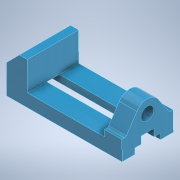
# Autodesk Inventor part: Parte2_Base
Saved by Autodesk Inventor 2021 (Build 250183000, 183)
## iProperties
Created: 2020-10-13
Part Number: Parte2_Base
Material: Steel, Carbon
Document SubType Name: Modeling
Designer: Alejandro Guevara
Density: 7.85 g/cm^3
Appearance: Sky Blue Dark
Author: Alejandro Guevara
Autodesk Inventor part; units mm, degrees
ref_plane "YZ Plane" through (0, 0, 0) normal (1, 0, 0) x (0, 1, 0)
ref_plane "XZ Plane" through (0, 0, 0) normal (0, 1, 0) x (-1, 0, 0)
ref_plane "XY Plane" through (0, 0, 0) normal (0, 0, 1) x (1, 0, 0)
sketch "Sketch1" plane through (0, 0, 0) normal (0, 0, 1) x (1, 0, 0)
  line L0 (-71.9595, -8.3565) -> (72.0387, -7.6433)
  line L1 (72.0387, -7.6433) -> (71.7812, 44.356)
  line L2 (71.7812, 44.356) -> (49.7815, 44.2471)
  line L3 (49.7815, 44.2471) -> (49.9598, 8.2475)
  line L4 (49.9598, 8.2475) -> (-46.0391, 7.7721)
  line L5 (-46.0391, 7.7721) -> (-46.2173, 43.7717)
  line L6 (-46.2173, 43.7717) -> (-56.2172, 43.7221)
  line L7 (-71.9595, -8.3565) -> (-71.9595, 27.7497)
  line L8 (-71.9595, 27.7497) -> (-56.2172, 43.7221)
  point P0 (0, 0)
  dimension "d0" = 144
  dimension "d1" = 52
  dimension "d2" = 22
  dimension "d3" = 36
  dimension "d4" = 96
  dimension "d5" = 36
  dimension "d6" = 10
  dimension "d8" = 72
  dimension "d9" = 16
  dimension "d10" = 8
  constraints: 18 end point, 4 perpendicular, 2 point on line, 1 vertical
  measures "d0" distance of L0.start L0.end
  measures "d1" distance of L0.end L1.end
  measures "d2" distance of L1.end L2.end
  measures "d3" distance of L2.end L3.end
  measures "d4" distance of L3.end L4.end
  measures "d5" distance of L4.end L5.end
  measures "d6" distance of L5.end L6.end
  measures "d8" distance from line of L1 point (0, 0)
  measures "d9" distance between parallel lines of L0 L4
  measures "d10" distance from line of L4 point (0, 0)
extrude "Extrusion1" add sketch "Sketch1" along normal blind 64
sketch "Sketch3" plane through (71.7812, 44.356, 64) normal (0.9999877, 0.0049523, 0) x (0, 0, -1)
  line L0 (64, -52) -> (64, 0) projected
  line L1 (0, -52) -> (0, 0) projected
  line L2 (48, -52) -> (48, -45)
  line L3 (40, -45) -> (40, -36)
  line L4 (48, -45) -> (40, -45)
  line L5 (40, -36) -> (32, -36)
  line L6 (64, -36) -> (0, -36) projected
  line L7 (16, -52) -> (16, -45)
  line L8 (24, -45) -> (24, -36)
  line L9 (16, -45) -> (24, -45)
  line L10 (24, -36) -> (32, -36)
  line L11 (16, -52) -> (48, -52)
  line L12 (64, -52) -> (0, -52) projected
  line L13 (64, -36) -> (64, 0) projected
  arc A0 (58.5136, -26.6786) -> (61, -28) centre (61, -25) ccw
  arc A1 (45.2611, -7.0477) -> (18.7389, -7.0477) centre (32, -16) ccw
  circle A2 centre (32, -16) radius 8
  line L14 (64, 0) -> (0, 0) projected
  line L15 (45.2611, -7.0477) -> (58.5136, -26.6786)
  line L16 (64, -28) -> (61, -28)
  line L17 (64, -15.8943) -> (0, -15.8943) projected
  arc A3 (3, -28) -> (5.4864, -26.6786) centre (3, -25) ccw
  line L18 (18.7389, -7.0477) -> (5.4864, -26.6786)
  line L19 (0, -28) -> (3, -28)
  line L20 (0, -36) -> (0, 0) projected
  line L21 (0, -28) -> (0, 0)
  line L22 (64, 0) -> (0, 0) projected
  line L23 (0, 0) -> (64, 0)
  line L24 (64, 0) -> (64, -28)
  point P0 (64, -44)
  point P1 (32, 0)
  point P2 (0, -28)
  point P3 (64, -28)
  dimension "d13" = 64
  dimension "d16" = 7
  dimension "d18" = 32
  dimension "d19" = 16
  dimension "d20" = 16
  dimension "d21" = 9
  dimension "d24" = 24
  dimension "d26" = 6
  dimension "d27" = 32
  dimension "d28" = 16
  dimension "d29" = 32
  dimension "d30" = 64
  constraints: 32 end point, 6 point on circle, 5 tangent, 4 centre point, 4 perpendicular, 2 collinear, 1 coincident, 1 midpoint, 1 point on line
  measures "d13" distance between parallel lines of L0 L1
  measures "d16" distance of L2.start L2.end
  measures "d18" distance between parallel lines of L2 L7
  measures "d19" distance between parallel lines of L3 L8
  measures "d20" distance from line of L0.start L2
  measures "d21" distance between parallel lines of L6 L9
  measures "d24" distance of L0.start L16.start
  measures "d26" diameter of A0
  measures "d27" diameter of A1
  measures "d28" diameter of A2
  measures "d29" distance from line of L1 A2.centre
  measures "d30" distance between parallel lines of L13 L1
extrude "Extrusion2" cut sketch "Sketch3" against normal through all contours L11 L7 L9 L8 L6 L5 L3 L4 L2
extrude "Extrusion3" cut sketch "Sketch3" against normal blind 22 contours L16 A0 L15 L17 L0 | L17 L15 A1 L14 L0 | A1 L18 L17 L1 L14 | L17 A2 | A2 L17 | L1 L17 L18 A3 L19
sketch "Sketch4" plane through (-45.9598, -8.2277, 64) normal (-0.0049523, 0.9999877, 0) x (0.9999877, 0.0049523, 0)
  line L0 (118, 16) -> (118, 0) projected
  line L1 (96, 0) -> (0, 0) projected
  circle A0 centre (80, 10) radius 3
  circle A1 centre (10, 10) radius 3
  line L2 (-40.7838, 32) -> (143.3901, 32)
  circle A2 centre (80, 54) radius 3
  circle A3 centre (10, 54) radius 3
  point P0 (46, 64)
  dimension "d35" = 6
  dimension "d37" = 6
  constraints: 4 centre point, 2 end point, 2 symmetric about line, 1 horizontal, 2 other
  measures "d35" diameter of A0
  measures "d37" diameter of A1
extrude "Extrusion4" cut sketch "Sketch4" along normal blind 15
equation "\"d8\" = 0.5 * d0"
equation "\"d10\" = 0.5 * d9"
equation "\"d29\" = 0.5 * d30"
body "Solid1"
